Autodesk Fusion 360 part; units mm, degrees
note: some values were not read from the file. Set by a fixed rule: which face or edge a step refers to.
(part 2 of 2)
sketch "Sketch19" plane through (0, -28, 0) normal (0, -1, 0) x (1, 0, 0)
  line L0 (187.5, 81) -> (160, 81)
  line L1 (160, 81) -> (160, 80.9937)
  spline S0 degree 3 poles (160, 80.9937) (150.3482, 80.8224) (141.2176, 80.4396) (132.8521, 79.8035) (122.3837, 79.0075) (113.1343, 77.8331) (105.3471, 76.0639) (100.6123, 74.9881) (96.4174, 73.7157) (92.6384, 71.9379) (90.0877, 70.738) (87.6935, 69.3141) (85.5066, 67.2576) (83.9716, 65.8142) (82.5316, 64.0162) (81.5103, 61.7976) (80.5939, 59.807) (80.0693, 57.4847) (80.0833, 55.2136) (80.0834, 55.1851) (80.0836, 55.1565) (80.0838, 55.128) knots -0.380217 -0.380217 -0.380217 -0.380217 -0.2899 -0.2899 -0.2899 -0.176878 -0.176878 -0.176878 -0.108156 -0.108156 -0.108156 -0.061771 -0.061771 -0.061771 -0.029213 -0.029213 -0.029213 0 0 0 0.00102 0.00102 0.00102 0.00102
  spline S1 degree 3 poles (80.0838, 55.128) (80.0844, 55.0995) (80.0851, 55.071) (80.0858, 55.0425) (80.0975, 54.5363) (80.134, 54.0286) (80.1955, 53.5241) (80.4774, 51.2077) (81.3112, 48.9949) (82.4288, 47.164) (83.7899, 44.9342) (85.5074, 43.2358) (87.3028, 41.8568) (89.687, 40.0255) (92.2561, 38.7039) (95.0386, 37.5637) (98.8082, 36.0189) (102.9997, 34.8321) (107.6808, 33.8168) (114.5551, 32.326) (122.4806, 31.2327) (131.2931, 30.4153) (139.5092, 29.6533) (148.4908, 29.1373) (158, 28.8289) knots -1.001016 -1.001016 -1.001016 -1.001016 -1 -1 -1 -0.993496 -0.993496 -0.993496 -0.963637 -0.963637 -0.963637 -0.927274 -0.927274 -0.927274 -0.878987 -0.878987 -0.878987 -0.813569 -0.813569 -0.813569 -0.717499 -0.717499 -0.717499 -0.627932 -0.627932 -0.627932 -0.627932
  line L2 (158, 28.8289) -> (158, 29)
  line L3 (158, 29) -> (187.5, 29)
  line L4 (187.5, 29) -> (187.5, 20)
  line L5 (187.5, 20) -> (176.1, 20)
  line L6 (176.1, 20) -> (173.9, 20)
  line L7 (160, 20) -> (160, 5)
  line L8 (160, 5) -> (5, 5)
  line L9 (5, 5) -> (5, 105)
  line L10 (5, 105) -> (160, 105)
  line L11 (160, 90) -> (173.9, 90)
  line L12 (173.9, 90) -> (176.1, 90)
  line L13 (187.5, 90) -> (187.5, 81)
  line L14 (190.0609, 2.4) -> (190, 33.4693)
  line L15 (190, 33.4693) -> (180.0334, 33.4693)
  spline S2 degree 3 poles (85.0834, 55.2015) (85.1068, 54.1955) (85.2621, 52.759) (86.4016, 50.2112) (87.0737, 48.9777) (89.9279, 45.9257) (92.1317, 44.3816) (100.5133, 40.4492) (107.8482, 38.6647) (136.8603, 33.9502) (164.5729, 33.5008) (180.0334, 33.4693) knots -9.827045 -9.827045 -9.827045 -9.827045 -8.213218 -8.213218 -7.416849 -7.416849 -6.408432 -6.408432 -4.638162 -4.638162 0 0 0 0
  spline S3 degree 3 poles (180.0619, 76.065) (166.0703, 76.1941) (150.913, 75.9958) (122.4781, 74.134) (110.7492, 72.5443) (96.8266, 68.5789) (93.9137, 67.0804) (90.5259, 65.0507) (89.1724, 63.956) (86.8287, 61.3733) (86.2047, 60.0899) (85.0703, 57.3337) (85.0806, 55.657) (85.0834, 55.2015) knots -0.389228 -0.389228 -0.389228 -0.389228 -0.329659 -0.329659 -0.267908 -0.267908 -0.229652 -0.229652 -0.187711 -0.187711 -0.136677 -0.136677 0 0 0 0
  line L16 (180.0619, 76.065) -> (190, 76.065)
  line L17 (190, 76.065) -> (190, 107.6)
  line L18 (190, 107.6) -> (2.4, 107.6)
  line L19 (2.4, 107.6) -> (2.4, 2.4)
  line L20 (2.4, 2.4) -> (190.0609, 2.4)
  line L21 (2.4, 107.6) -> (2.4, 102.6)
  line L22 (2.4, 102.6) -> (6.65, 102.6)
  line L23 (173.9, 20) -> (160, 20)
  line L24 (160, 105) -> (160, 90)
  line L25 (176.1, 90) -> (187.5, 90)
  line L26 (2.4, 2.4) -> (7.4, 2.4)
  line L27 (7.4, 2.4) -> (7.4, 7.4)
  line L28 (190, 107.6) -> (185, 107.6)
  line L29 (185, 107.6) -> (185, 102.6)
  line L30 (190.0609, 2.4) -> (185.0609, 2.4)
  line L31 (185.0609, 2.4) -> (185.0609, 7.4)
  circle A0 centre (185, 102.6) radius 0.75
  circle A1 centre (185.0609, 7.4) radius 0.75
  circle A2 centre (7.4, 7.4) radius 0.75
  circle A3 centre (7.4, 102.6) radius 0.75
  dimension "d350" = 5
  dimension "d358" = 5
  dimension "d359" = 5
  dimension "d364" = 5
  dimension "d365" = 5
  dimension "d366" = 5
  dimension "d367" = 5
  dimension "d372" = 1.5
  dimension "d373" = 1.5
  dimension "d374" = 1.5
  dimension "d375" = 1.5
  measures "d350" distance of L18.end L21.end
  measures "d358" distance of L19.end L26.end
  measures "d359" distance of L26.end L27.end
  measures "d364" distance of L17.end L28.end
  measures "d365" distance of L28.end L29.end
  measures "d366" distance of L14.start L30.end
  measures "d367" distance of L30.end L31.end
  measures "d372" diameter of A0
  measures "d373" diameter of A1
  measures "d374" diameter of A2
  measures "d375" diameter of A3
sketch "Sketch20" plane through (0, 0, 5) normal (0, 0, 1) x (1, 0, 0)
  line L0 (8, 0) -> (5, 0)
  line L1 (5, 0) -> (5, -28)
  line L2 (5, -28) -> (160, -28)
  line L3 (160, -28) -> (160, 0)
  line L4 (160, 0) -> (72, 0)
  line L5 (72, 0) -> (8, 0)
  line L6 (5, -28) -> (5, -18)
  line L7 (72, 0) -> (72, -12)
  line L8 (72, -12) -> (72, 0)
  line L9 (8, 0) -> (8, -12)
  line L10 (8, -12) -> (8, 0)
  dimension "d355" = 10
  measures "d355" distance of L1.end L6.end
loft "Loft2" add profiles "Sketch18" section 1 point at (5, -18, 5) section 2 contours L9 L10 L28 L29 L30 L31 bodies 2
loft "Loft3" add profiles "Sketch18" section 1 point at (5, -18, 105) section 2 contours L10 L11 L24 L25 L26 L27 bodies 2
extrude "Extrude43" cut sketch "Sketch19" against normal blind 4 contours A0 | A1 | A2 | A3 bodies 2
extrude "Extrude42" cut 2 faces at (205.0673, -28, 8.4358) (204.9327, -28, 101.5642) along direction (0, -1, 0) blind 3 on bodies 2 bodies 2
sketch "Sketch26" plane through (0, 0.7, 0) normal (0, 1, 0) x (-1, 0, 0)
  line L0 (-180.0334, 33.4693) -> (-220, 33.4693)
  line L1 (-220, 33.4693) -> (-220, 0)
  line L2 (-220, 0) -> (0, 0)
  line L3 (0, 0) -> (0, 110)
  line L4 (0, 110) -> (-220, 110)
  line L5 (-220, 110) -> (-220, 76.065)
  line L6 (-220, 76.065) -> (-180.0619, 76.065)
  spline S0 degree 3 poles (-180.0619, 76.065) (-159.1795, 76.2576) (-139.8387, 75.6828) (-124.2368, 73.9979) (-115.6615, 73.0718) (-108.2229, 71.8213) (-102.1502, 70.0947) (-98.213, 68.9753) (-94.844, 67.6751) (-92.0221, 65.9426) (-90.1417, 64.7881) (-88.4752, 63.4272) (-87.1878, 61.6436) (-86.1381, 60.1892) (-85.3752, 58.4147) (-85.1541, 56.5302) (-85.104, 56.1036) (-85.0805, 55.6734) (-85.0832, 55.2442) (-85.0832, 55.23) (-85.0833, 55.2157) (-85.0834, 55.2015) knots -0.440962 -0.440962 -0.440962 -0.440962 -0.255755 -0.255755 -0.255755 -0.153959 -0.153959 -0.153959 -0.087961 -0.087961 -0.087961 -0.04398 -0.04398 -0.04398 -0.008119 -0.008119 -0.008119 0 0 0 0.00051 0.00051 0.00051 0.00051
  spline S1 degree 3 poles (-85.0834, 55.2015) (-85.0838, 55.1872) (-85.0841, 55.173) (-85.0844, 55.1587) (-85.1283, 53.2729) (-85.7115, 51.4171) (-86.6378, 49.8664) (-87.8395, 47.8546) (-89.5287, 46.3185) (-91.4514, 45.0322) (-94.4377, 43.0345) (-98.0815, 41.5688) (-102.3978, 40.3015) (-109.8672, 38.1085) (-119.3843, 36.5903) (-130.4817, 35.5147) (-144.8663, 34.1205) (-161.8701, 33.5063) (-180.0283, 33.4693) (-180.03, 33.4693) (-180.0317, 33.4693) (-180.0334, 33.4693) knots -1.000508 -1.000508 -1.000508 -1.000508 -1 -1 -1 -0.964386 -0.964386 -0.964386 -0.918178 -0.918178 -0.918178 -0.846413 -0.846413 -0.846413 -0.722224 -0.722224 -0.722224 -0.561247 -0.561247 -0.561247 -0.561232 -0.561232 -0.561232 -0.561232
  line L7 (-195, 105) -> (-195, 81.065)
  line L8 (-195, 81.065) -> (-215, 81.065)
  line L9 (-215, 81.065) -> (-215, 105)
  line L10 (-215, 105) -> (-195, 105)
  line L11 (-195, 5) -> (-215, 5)
  line L12 (-215, 5) -> (-215, 28.4693)
  line L13 (-215, 28.4693) -> (-195, 28.4693)
  line L14 (-195, 28.4693) -> (-195, 5)
  line L15 (13, 68.75) -> (0, 89.375)
  line L16 (0, 20.625) -> (0, 0)
  line L17 (13, 41.25) -> (0, 20.625)
  line L18 (13, 41.25) -> (13, 68.75)
  line L19 (0, 89.375) -> (0, 20.625)
  line L20 (-80.0868, 65) -> (-62.0868, 65)
  line L21 (-62.0868, 65) -> (-62.0868, 45)
  line L22 (-62.0868, 45) -> (-80.0868, 45)
  line L23 (-80.0868, 45) -> (-80.0868, 55)
  spline S2 degree 3 poles (-80.0868, 55) (-80.0864, 55.0142) (-80.0861, 55.0283) (-80.0858, 55.0425) (-80.0851, 55.071) (-80.0844, 55.0995) (-80.0838, 55.128) knots 0.999818 0.999818 0.999818 0.999818 1 1 1 1.001016 1.001016 1.001016 1.001016
  spline S3 degree 3 poles (-80.0838, 55.128) (-80.0836, 55.1565) (-80.0834, 55.1851) (-80.0833, 55.2136) (-80.0824, 55.354) (-80.0836, 55.4946) (-80.0868, 55.6354) knots -0.00102 -0.00102 -0.00102 -0.00102 0 0 0 0.001806 0.001806 0.001806 0.001806
  line L24 (-80.0868, 55.6354) -> (-80.0868, 65)
extrude "Extrude47" add sketch "Sketch26" against normal blind 32.7 contours L3 L15 L17 L18 L19 bodies 2
sketch "Sketch27" plane through (-13, 0, 0) normal (-1, 0, 0) x (0, 0, 1)
  line L0 (68.75, 0.7) -> (41.25, 0.7)
  line L1 (41.25, 0.7) -> (41.25, -32)
  line L2 (41.25, -32) -> (68.75, -32)
  line L3 (68.75, -32) -> (68.75, 0.7)
  circle A0 centre (55, -15.65) radius 8
  dimension "d433" = 16
  measures "d433" diameter of A0
extrude "Extrude48" cut sketch "Sketch27" against normal blind 18 contours A0 bodies 2
sketch "Sketch28" plane through (5, 0, 0) normal (1, 0, 0) x (0, 0, -1)
  circle A0 centre (-55, -15.65) radius 8
  line L0 (-105, -18) -> (-97.5, -28)
  line L1 (-97.5, -28) -> (-12.5, -28)
  line L2 (-12.5, -28) -> (-5, -18)
  line L3 (-5, -18) -> (-5, 0)
  line L4 (-5, 0) -> (-8, 0)
  line L5 (-8, 0) -> (-102, 0)
  line L6 (-102, 0) -> (-105, 0)
  line L7 (-105, 0) -> (-105, -18)
  line L8 (-55, -15.65) -> (-40, -15.65)
  line L9 (-40, -15.65) -> (-40, -25.65)
  line L10 (-70, -25.65) -> (-70, -5.65)
  line L11 (-70, -5.65) -> (-40, -5.65)
  line L12 (-40, -5.65) -> (-40, -25.65)
  line L13 (-40, -25.65) -> (-70, -25.65)
  line L14 (-8, 0) -> (-8, -12)
  line L15 (-8, -12) -> (-8, 0)
  line L16 (-102, 0) -> (-102, -12)
  line L17 (-102, -12) -> (-102, 0)
  dimension "d436" = 15
  dimension "d437" = 10
  dimension "d438" = 30
  dimension "d439" = 20
  measures "d436" distance of A0.centre L8.end
  measures "d437" distance of L8.end L9.end
  measures "d438" distance of L9.end L10.start
  measures "d439" distance of L9.end L11.end
extrude "Extrude49" cut sketch "Sketch28" against normal blind 13 contours L9 L10 L11 L12 L13 bodies 2
fillet "Fillet4" radius 10 2 edges at (-13, -15.65, 41.25) (-13, -15.65, 68.75) on bodies 2
fillet "Fillet5" radius 49 2 edges at (0, -15.65, 20.625) (0, -15.65, 89.375) on bodies 2
fillet "Fillet6" radius 45 1 edges at (5, -15.65, 40) on bodies 2
sketch "Sketch29" plane through (0, 0.7, 0) normal (0, 1, 0) x (-1, 0, 0)
  arc A0 (13, 65.8614) -> (11.4598, 71.1937) centre (3, 65.8614) ccw
  line L0 (11.4598, 71.1937) -> (7.5472, 77.4011)
  arc A1 (0, 103.5289) -> (7.5472, 77.4011) centre (49, 103.5289) ccw
  line L1 (0, 103.5289) -> (0, 110)
  line L2 (0, 110) -> (-220, 110)
  line L3 (-220, 110) -> (-220, 76.065)
  line L4 (-220, 76.065) -> (-180.0619, 76.065)
  spline S0 degree 3 poles (-180.0619, 76.065) (-159.1795, 76.2576) (-139.8387, 75.6828) (-124.2368, 73.9979) (-115.6615, 73.0718) (-108.2229, 71.8213) (-102.1502, 70.0947) (-98.213, 68.9753) (-94.844, 67.6751) (-92.0221, 65.9426) (-90.1417, 64.7881) (-88.4752, 63.4272) (-87.1878, 61.6436) (-86.1381, 60.1892) (-85.3752, 58.4147) (-85.1541, 56.5302) (-85.104, 56.1036) (-85.0805, 55.6734) (-85.0832, 55.2442) (-85.0832, 55.23) (-85.0833, 55.2157) (-85.0834, 55.2015) knots -0.440962 -0.440962 -0.440962 -0.440962 -0.255755 -0.255755 -0.255755 -0.153959 -0.153959 -0.153959 -0.087961 -0.087961 -0.087961 -0.04398 -0.04398 -0.04398 -0.008119 -0.008119 -0.008119 0 0 0 0.00051 0.00051 0.00051 0.00051
  spline S1 degree 3 poles (-85.0834, 55.2015) (-85.0838, 55.1872) (-85.0841, 55.173) (-85.0844, 55.1587) (-85.1283, 53.2729) (-85.7115, 51.4171) (-86.6378, 49.8664) (-87.8395, 47.8546) (-89.5287, 46.3185) (-91.4514, 45.0322) (-94.4377, 43.0345) (-98.0815, 41.5688) (-102.3978, 40.3015) (-109.8672, 38.1085) (-119.3843, 36.5903) (-130.4817, 35.5147) (-144.8663, 34.1205) (-161.8701, 33.5063) (-180.0283, 33.4693) (-180.03, 33.4693) (-180.0317, 33.4693) (-180.0334, 33.4693) knots -1.000508 -1.000508 -1.000508 -1.000508 -1 -1 -1 -0.964386 -0.964386 -0.964386 -0.918178 -0.918178 -0.918178 -0.846413 -0.846413 -0.846413 -0.722224 -0.722224 -0.722224 -0.561247 -0.561247 -0.561247 -0.561232 -0.561232 -0.561232 -0.561232
  line L5 (-180.0334, 33.4693) -> (-220, 33.4693)
  line L6 (-220, 33.4693) -> (-220, 0)
  line L7 (-220, 0) -> (0, 0)
  line L8 (0, 0) -> (0, 6.4711)
  arc A2 (7.5472, 32.5989) -> (0, 6.4711) centre (49, 6.4711) ccw
  line L9 (7.5472, 32.5989) -> (11.4598, 38.8063)
  arc A3 (11.4598, 38.8063) -> (13, 44.1386) centre (3, 44.1386) ccw
  line L10 (13, 44.1386) -> (13, 65.8614)
  line L11 (-80.0868, 65) -> (-62.0868, 65)
  line L12 (-62.0868, 65) -> (-62.0868, 45)
  line L13 (-62.0868, 45) -> (-80.0868, 45)
  line L14 (-80.0868, 45) -> (-80.0868, 55)
  spline S2 degree 3 poles (-80.0868, 55) (-80.0864, 55.0142) (-80.0861, 55.0283) (-80.0858, 55.0425) (-80.0851, 55.071) (-80.0844, 55.0995) (-80.0838, 55.128) knots 0.999818 0.999818 0.999818 0.999818 1 1 1 1.001016 1.001016 1.001016 1.001016
  spline S3 degree 3 poles (-80.0838, 55.128) (-80.0836, 55.1565) (-80.0834, 55.1851) (-80.0833, 55.2136) (-80.0824, 55.354) (-80.0836, 55.4946) (-80.0868, 55.6354) knots -0.00102 -0.00102 -0.00102 -0.00102 0 0 0 0.001806 0.001806 0.001806 0.001806
  line L15 (-80.0868, 55.6354) -> (-80.0868, 65)
  line L16 (-195, 5) -> (-215, 5)
  line L17 (-215, 5) -> (-215, 28.4693)
  line L18 (-215, 28.4693) -> (-195, 28.4693)
  line L19 (-195, 28.4693) -> (-195, 5)
  line L20 (-195, 105) -> (-195, 81.065)
  line L21 (-195, 81.065) -> (-215, 81.065)
  line L22 (-215, 81.065) -> (-215, 105)
  line L23 (-215, 105) -> (-195, 105)
  line L24 (80.8868, -65.8) -> (61.2868, -65.8)
  line L25 (80.0868, -67.8) -> (59.2868, -67.8)
  line L26 (61.2868, -44.2) -> (80.8868, -44.2)
  line L27 (80.0868, -65) -> (62.0868, -65)
  line L28 (82.0868, -67) -> (60.0868, -67)
  line L29 (62.0868, -45) -> (80.0868, -45)
  line L30 (60.0868, -43) -> (82.0868, -43)
  line L31 (60.0868, -67) -> (60.0868, -43)
  line L32 (61.2868, -65.8) -> (61.2868, -44.2)
  line L33 (59.2868, -67.8) -> (59.2868, -42.2)
  line L34 (62.0868, -65) -> (62.0868, -45)
  line L35 (80.0868, -42.2) -> (86.8661, -42.2)
  line L36 (80.0868, -45) -> (80.0868, -65)
  line L37 (59.2868, -42.2) -> (80.0868, -42.2)
  line L38 (80.0868, -55) -> (80.0868, -65)
  line L39 (80.0839, -55) -> (80.0868, -55)
  line L40 (80.0868, -67.8) -> (86.1046, -67.8)
  line L41 (80.8868, -44.2) -> (80.8868, -65.8)
  line L42 (82.0868, -43) -> (82.0868, -67)
  line L43 (-60.0868, 43) -> (-82.0868, 43)
  line L44 (-82.0868, 43) -> (-82.0868, 67)
  line L45 (-82.0868, 67) -> (-60.0868, 67)
  line L46 (-62.0868, 45) -> (-62.0868, 43)
  line L47 (-62.0868, 45) -> (-60.0868, 45)
  line L48 (-60.0868, 45) -> (-60.0868, 43)
  line L49 (-60.0868, 67) -> (-60.0868, 43)
  point P0 (80.0838, -55.128)
  point P1 (85.0834, -55.2015)
  dimension "d452" = 2
  dimension "d453" = 0.8
  dimension "d454" = 2.8
  dimension "d455" = 10
  dimension "d456" = 18
  dimension "d457" = 20
  dimension "d460" = 24
  dimension "d461" = 22
  measures "d455" distance of L38.start L27.start
  measures "d456" distance of L27.start L27.end
  measures "d457" distance of L29.end L27.start
  measures "d460" distance of L43.start L45.end
  measures "d461" distance of L43.start L43.end
extrude "Extrude53" cut sketch "Sketch29" against normal blind 1 contours L43 L44 L45 L46 L47 L49 | L43 L46 L47 L48 L49 bodies 1 2
fillet "Fillet7" radius 45 1 edges at (5, -15.65, 70) on bodies 2
extrude "Extrude54" cut 6 faces at (220, 0.2333, 98.6883) (220, -13.1, 98.6883) (220, -15.5333, 72.8282) (220, 0.2333, 22.3129) (220, -13.1, 11.1564) (220, -15.5333, 36.6778) along direction (-1, 0, 0) blind 3 on bodies 2 bodies 2
combine "Combine1" operation add target body 2 tool bodies 1
